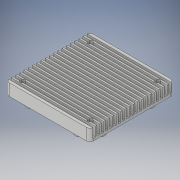
# Autodesk Inventor part: 10_Cube_sampleholder
Saved by Autodesk Inventor 2019 (Build 230136000, 136)
## iProperties
Created: 2018-07-23
Part Number: 10_Cube_sampleholder
Material: Generisch
Document SubType Name: Modeling
Designer: diederichbenedict
Density: 1 g/cm^3
Appearance: Vorgabe
Author: diederichbenedict
Autodesk Inventor part; units mm, degrees
ref_plane "YZ Plane" through (0, 0, 0) normal (1, 0, 0) x (0, 1, 0)
ref_plane "XZ Plane" through (0, 0, 0) normal (0, 1, 0) x (-1, 0, 0)
ref_plane "Arbeitsebene1" through (0, 0, 0) normal (0, 0, 1) x (1, 0, 0)
sketch "Skizze1" plane through (0, 0, 0) normal (0, 0, 1) x (1, 0, 0)
  arc A0 (-22.9, 24.9) -> (-24.9, 22.9) centre (-22.9, 22.9) ccw projected
  line L0 (-24.9, 22.9) -> (-24.9, -22.9) projected
  arc A1 (-24.9, -22.9) -> (-22.9, -24.9) centre (-22.9, -22.9) ccw projected
  line L1 (-22.9, -24.9) -> (22.9, -24.9) projected
  arc A2 (22.9, -24.9) -> (24.9, -22.9) centre (22.9, -22.9) ccw projected
  line L2 (24.9, -22.9) -> (24.9, 22.9) projected
  arc A3 (24.9, 22.9) -> (22.9, 24.9) centre (22.9, 22.9) ccw projected
  line L3 (22.9, 24.9) -> (-22.9, 24.9) projected
  circle A4 centre (20, 20) radius 1.6 projected
  circle A5 centre (-20, -20) radius 1.6 projected
  circle A6 centre (20, -20) radius 1.6 projected
  circle A7 centre (-20, 20) radius 1.6 projected
  arc A8 (6.7383, -21.066) -> (8.3017, -21.066) centre (7.52, -20.62) ccw projected
  line L4 (6.7383, -21.066) -> (-6.9383, -21.066) projected
  arc A9 (-8.5017, -21.066) -> (-6.9383, -21.066) centre (-7.72, -20.62) ccw projected
  line L5 (-8.5017, -21.066) -> (-17.9, -21.066) projected
  line L6 (-17.9, -21.066) -> (-17.9, 21.066) projected
  line L7 (-17.9, 21.066) -> (17.9, 21.066) projected
  line L8 (17.9, 21.066) -> (17.9, 12) projected
  arc A10 (14.9, 9) -> (17.9, 12) centre (14.9, 12) ccw projected
  line L9 (14.5, 9) -> (14.9, 9) projected
  arc A11 (14.5, 9) -> (11.5, 6) centre (14.5, 6) ccw projected
  line L10 (11.5, -6) -> (11.5, 6) projected
  arc A12 (11.5, -6) -> (14.5, -9) centre (14.5, -6) ccw projected
  line L11 (14.9, -9) -> (14.5, -9) projected
  arc A13 (17.9, -12) -> (14.9, -9) centre (14.9, -12) ccw projected
  line L12 (17.9, -12) -> (17.9, -21.066) projected
  line L13 (17.9, -21.066) -> (8.3017, -21.066) projected
  arc A14 (13.4381, 5.6873) -> (13.3881, 5.2) centre (15.7881, 5.2) ccw projected
  line L14 (13.4381, 5.6873) -> (13.4381, 7.6) projected
  line L15 (13.4381, 7.6) -> (15.7881, 7.6) projected
  arc A15 (18.1881, 5.2) -> (15.7881, 7.6) centre (15.7881, 5.2) ccw projected
  line L16 (18.1881, 5.2) -> (18.1881, -5.2) projected
  arc A16 (15.7881, -7.6) -> (18.1881, -5.2) centre (15.7881, -5.2) ccw projected
  line L17 (15.7881, -7.6) -> (13.4381, -7.6) projected
  line L18 (13.4381, -7.6) -> (13.4381, -5.6873) projected
  arc A17 (13.3881, -5.2) -> (13.4381, -5.6873) centre (15.7881, -5.2) ccw projected
  line L19 (13.3881, -5.2) -> (13.3881, 5.2) projected
  line L20 (17.9, 21.066) -> (17.9, -21.066)
  point P0 (0, 0)
  constraints: 2 end point, 1 vertical
extrude "Extrusion1" add sketch "Skizze1" along normal blind 7 contours L3 A3 L2 A2 L1 A1 L0 A0 | A4 | A5 | A6 | A7 | L4 A9 L5 L6 L7 L8 A10 L9 A11 L10 A12 L11 A13 L12 L13 A8 | A13 L11 A12 L10 A11 L9 A10 L20 A15 L15 L14 A14 L19 A17 L18 L17 A16 | L20 A15 L16 A16 | A16 L17 L18 A17 L19 A14 L14 L15 A15 L20
sketch "Skizze2" plane through (0, 0, 7) normal (0, 0, 1) x (1, 0, 0)
  circle A0 centre (-20, 20) radius 1.6 projected
  circle A1 centre (20, 20) radius 1.6 projected
  circle A2 centre (20, -20) radius 1.6 projected
  circle A3 centre (-20, -20) radius 1.6 projected
  line L0 (24.9, -22.9) -> (24.9, 22.9) projected
  line L1 (-24.9, 0.75) -> (24.9, 0.75)
  line L2 (24.9, 0.75) -> (24.9, -0.75)
  line L3 (24.9, -0.75) -> (-24.9, -0.75)
  line L4 (-24.9, -0.75) -> (-24.9, 0.75)
  line L5 (-24.9, 0.75) -> (24.9, -0.75) construction
  line L6 (24.9, 0.75) -> (-24.9, -0.75) construction
  point P0 (0, 0)
  dimension "d2" = 1.5
  constraints: 12 end point, 2 midpoint, 2 parallel, 1 horizontal, 1 perpendicular, 1 point on line
  measures "d2" distance of L1.end L2.end
extrude "Extrusion2" cut sketch "Skizze2" against normal blind 5.5 contours L3 L4 L1 L0
pattern_linear "Rechteckige Anordnung1" count 10 spacing 2.5 along (0, -1, 0) count 10 spacing 2.5 along (0, 1, 0) of "Extrusion2"
sketch "Skizze3" plane through (0, 0, 7) normal (0, 0, 1) x (1, 0, 0)
  circle A0 centre (-20, -20) radius 1.6 projected
  line L0 (18.8686, -21.1314) -> (18.4, -21.6) projected
  arc A1 (22.9, -19.2319) -> (19.2319, -22.9) centre (20, -20) ccw projected
  circle A2 centre (20, 20) radius 1.6 projected
  circle A3 centre (-20, 20) radius 1.6 projected
  point P0 (0, 0)
hole "Bohrung1" at (-20, 20, 7) at (20, 20, 7) at (20, -20, 7) at (-20, -20, 7) direction (0, 0, -1) diameter 2.7 end through all
sketch "Sketch4" plane through (0, 0, 0) normal (0, 0, -1) x (-1, 0, 0)
  circle A0 centre (-20, -20) radius 1.35 construction
  circle A1 centre (20, 20) radius 1.35 construction
  circle A2 centre (-20, 20) radius 1.35 construction
  circle A3 centre (20, -20) radius 1.35 construction
  arc A4 (24.9, 22.9) -> (22.9, 24.9) centre (22.9, 22.9) ccw construction
  line L0 (22.9, 24.9) -> (-22.9, 24.9) construction
  arc A5 (-22.9, 24.9) -> (-24.9, 22.9) centre (-22.9, 22.9) ccw construction
  line L1 (-24.9, 22.9) -> (-24.9, -22.9) construction
  arc A6 (-24.9, -22.9) -> (-22.9, -24.9) centre (-22.9, -22.9) ccw construction
  line L2 (-22.9, -24.9) -> (22.9, -24.9) construction
  arc A7 (22.9, -24.9) -> (24.9, -22.9) centre (22.9, -22.9) ccw construction
  line L3 (24.9, -22.9) -> (24.9, 22.9) construction
  line L4 (35.4399, 0) -> (-35.4399, 0) construction
  line L5 (0, -35.4399) -> (0, 35.4399) construction
  circle A8 centre (21, 0.2) radius 2.5 construction
  circle A9 centre (-0.4, -21) radius 2.5 construction
  line L6 (-4.8804, 23.8709) -> (-4.8804, 25) construction
  line L7 (-4.8804, 25) -> (-23, 25) construction
  arc A10 (-23, 25) -> (-25, 23) centre (-23, 23) ccw construction
  line L8 (-25, 5.0901) -> (-25, 23) construction
  line L9 (-25, 5.0901) -> (-23.8731, 5.0901) construction
  arc A11 (-23.8731, 5.0901) -> (-23.4716, 5.4179) centre (-23.8731, 5.4998) ccw construction
  arc A12 (-19.3339, 5) -> (-23.4716, 5.4179) centre (-21.4238, 5) ccw construction
  line L10 (-19.3339, 5) -> (-19.3339, -4.7986) construction
  arc A13 (-23.4417, -5.341) -> (-19.3339, -4.7986) centre (-21.397, -5) ccw construction
  line L11 (-23.4417, -5.341) -> (-23.4722, -5.2203) construction
  arc A14 (-23.4722, -5.2203) -> (-23.8709, -4.8804) centre (-23.8777, -5.2921) ccw construction
  line L12 (-23.8709, -4.8804) -> (-25, -4.8804) construction
  line L13 (-25, -23) -> (-25, -4.8804) construction
  arc A15 (-25, -23) -> (-23, -25) centre (-23, -23) ccw construction
  line L14 (-23, -25) -> (-5, -25) construction
  line L15 (-5, -25) -> (-5, -26.0505) construction
  arc A16 (-5.4, -26.5404) -> (-5, -26.0505) centre (-5.5, -26.0505) ccw construction
  arc A17 (-5.4, -26.5404) -> (-5, -30.5) centre (-5, -28.5) ccw construction
  line L16 (-5, -30.5) -> (5, -30.5) construction
  arc A18 (5, -30.5) -> (5.4, -26.5404) centre (5, -28.5) ccw construction
  arc A19 (5, -26.0505) -> (5.4, -26.5404) centre (5.5, -26.0505) ccw construction
  line L17 (5, -26.0505) -> (5, -25) construction
  line L18 (5, -25) -> (23, -25) construction
  arc A20 (23, -25) -> (25, -23) centre (23, -23) ccw construction
  line L19 (25, -5) -> (25, -23) construction
  line L20 (25, -5) -> (26.0505, -5) construction
  arc A21 (26.5404, -5.4) -> (26.0505, -5) centre (26.0505, -5.5) ccw construction
  arc A22 (26.5404, -5.4) -> (30.5, -5) centre (28.5, -5) ccw construction
  line L21 (30.5, -5) -> (30.5, 5) construction
  arc A23 (30.5, 5) -> (26.5404, 5.4) centre (28.5, 5) ccw construction
  arc A24 (26.0505, 5) -> (26.5404, 5.4) centre (26.0505, 5.5) ccw construction
  line L22 (26.0505, 5) -> (25, 5) construction
  line L23 (25, 23) -> (25, 5) construction
  arc A25 (25, 23) -> (23, 25) centre (23, 23) ccw construction
  line L24 (23, 25) -> (5.0901, 25) construction
  line L25 (5.0901, 25) -> (5.0901, 23.8731) construction
  arc A26 (5.0901, 23.8731) -> (5.4179, 23.4716) centre (5.4998, 23.8731) ccw construction
  arc A27 (5, 19.3339) -> (5.4179, 23.4716) centre (5, 21.4238) ccw construction
  line L26 (5, 19.3339) -> (-4.7986, 19.3339) construction
  arc A28 (-5.341, 23.4417) -> (-4.7986, 19.3339) centre (-5, 21.397) ccw construction
  line L27 (-5.341, 23.4417) -> (-5.2203, 23.4722) construction
  arc A29 (-5.2203, 23.4722) -> (-4.8804, 23.8709) centre (-5.2921, 23.8777) ccw construction
  line L28 (15, 17) -> (-15, 17) construction
  arc A30 (17, 15) -> (15, 17) centre (15, 15) ccw construction
  line L29 (17, 15) -> (17, -15) construction
  arc A31 (15, -17) -> (17, -15) centre (15, -15) ccw construction
  line L30 (15, -17) -> (-15, -17) construction
  arc A32 (-17, -15) -> (-15, -17) centre (-15, -15) ccw construction
  line L31 (-17, -15) -> (-17, 15) construction
  arc A33 (-15, 17) -> (-17, 15) centre (-15, 15) ccw construction
  circle A34 centre (-20, 20) radius 2.425 construction
  circle A35 centre (-14.5, 20.8) radius 2.65 construction
  circle A36 centre (-20.8, 14.5) radius 2.65 construction
  circle A37 centre (-20, -20) radius 2.425 construction
  circle A38 centre (-14.5, -20.8) radius 2.65 construction
  circle A39 centre (-20.8, -14.5) radius 2.65 construction
  circle A40 centre (20, 20) radius 2.425 construction
  circle A41 centre (14.5, 20.8) radius 2.65 construction
  circle A42 centre (20.8, 14.5) radius 2.65 construction
  circle A43 centre (20.8, -14.5) radius 2.65 construction
  circle A44 centre (14.5, -20.8) radius 2.65 construction
  circle A45 centre (20, -20) radius 2.425 construction
  circle A46 centre (-14.5, 20.8) radius 2.4
  circle A47 centre (14.5, 20.8) radius 2.4
  circle A48 centre (20.8, 14.5) radius 2.4
  circle A49 centre (20.8, -14.5) radius 2.4
  circle A50 centre (14.5, -20.8) radius 2.4
  circle A51 centre (-14.5, -20.8) radius 2.4
  circle A52 centre (-20.8, -14.5) radius 2.4
  circle A53 centre (-20.8, 14.5) radius 2.4
  point P0 (-0.4, 0.2)
  dimension "d19" = 0.25
  dimension "d20" = 0.25
  dimension "d21" = 0.25
  dimension "d22" = 0.25
  dimension "d23" = 0.25
  dimension "d24" = 0.25
  dimension "d25" = 0.25
  dimension "d26" = 0.25
  constraints: 52 end point, 48 point on circle, 46 centre point, 8 other
  measures "d19" radial gap between concentric circles of A35 A46
  measures "d20" radial gap between concentric circles of A41 A47
  measures "d21" radial gap between concentric circles of A42 A48
  measures "d22" radial gap between concentric circles of A43 A49
  measures "d23" radial gap between concentric circles of A44 A50
  measures "d24" radial gap between concentric circles of A38 A51
  measures "d25" radial gap between concentric circles of A39 A52
  measures "d26" radial gap between concentric circles of A36 A53
extrude "Extrusion3" add sketch "Sketch4" along normal blind 2.4
equation "\"d20\" = d19"
equation "\"d21\" = d19"
equation "\"d22\" = d19"
equation "\"d23\" = d19"
equation "\"d24\" = d19"
equation "\"d25\" = d19"
equation "\"d26\" = d19"
